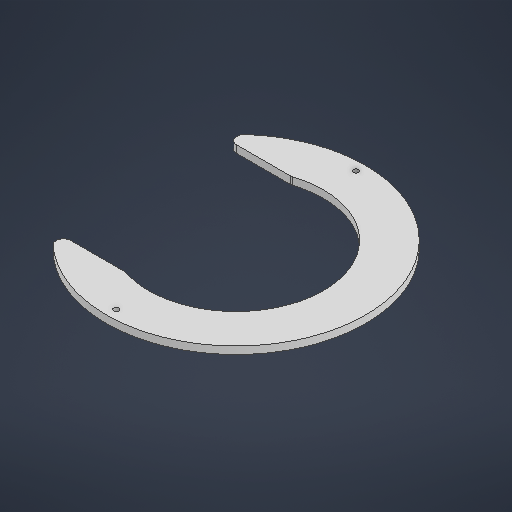
# Autodesk Inventor part: Cylinder Segment Holder
Saved by Autodesk Inventor 2025 (Build 290162000, 162)
## iProperties
Created: 2025-02-13
Part Number: Cylinder Segment Holder
Material: Generic
Document SubType Name: Modeling
Designer: mayhe
Density: 1 g/cm^3
Appearance: Default
Author: mayhe
Autodesk Inventor part; units mm, degrees
ref_plane "YZ Plane" through (0, 0, 0) normal (1, 0, 0) x (0, 1, 0)
ref_plane "XZ Plane" through (0, 0, 0) normal (0, 1, 0) x (-1, 0, 0)
ref_plane "XY Plane" through (0, 0, 0) normal (0, 0, 1) x (1, 0, 0)
sketch "Sketch1" plane through (0, 0, 0) normal (0, 1, 0) x (-1, 0, 0)
  circle A0 centre (0, 0) radius 59
  circle A1 centre (0, 0) radius 81
  circle A2 centre (0, 0) radius 87.5
  circle A3 centre (0, 81) radius 1.75
  circle A4 centre (0, -81) radius 1.75
  line L0 (90, -56) -> (15, -56)
  line L1 (10, -51) -> (10, 51)
  line L2 (15, 56) -> (90, 56)
  line L3 (90, 56) -> (90, -56)
  line L4 (90, -56) -> (10, 56) construction
  line L5 (10, -56) -> (90, 56) construction
  arc A5 (10, -51) -> (15, -56) centre (15, -51) ccw
  arc A6 (15, 56) -> (10, 51) centre (15, 51) ccw
  point P0 (50, 0)
  point P1 (90, 0)
  point P2 (10, 0)
  point P3 (60, -54.4151)
  point P4 (60, 54.4151)
  point P5 (80, 35.4436)
  point P6 (80, -35.4436)
  point P7 (67.2328, 56)
  point P8 (67.2328, -56)
  dimension "d0" = 118
  dimension "d1" = 162
  dimension "d2" = 175
  dimension "d3" = 3.5
  dimension "d4" = 3.5
  dimension "d7" = 112
  dimension "d9" = 80
  dimension "d10" = 10
  dimension "d11" = 5
  constraints: 12 end point, 7 centre point, 6 point on circle, 4 midpoint, 4 point on line, 4 tangent, 3 coincident, 2 parallel, 1 equal radius, 1 horizontal, 1 perpendicular
  measures "d0" diameter of A0
  measures "d1" diameter of A1
  measures "d2" diameter of A2
  measures "d3" diameter of A3
  measures "d4" diameter of A4
  measures "d7" distance of L4.end L5.start
  measures "d9" distance of L4.end L2.end
  measures "d10" distance of point (0, 0) point (10, 0)
  measures "d11" radius of A5
extrude "Extrusion1" add sketch "Sketch1" along normal blind 5 contours A0 L0 A1 A4 A3 L2 | A1 A3 A4 L0 A2 L2
fillet "Fillet1" radius 5 4 edges at (-67.2328, 2.5, -56) (-67.2328, 2.5, 56) (-18.5742, 2.5, -56) (-18.5742, 2.5, 56)
body "Solid1"
